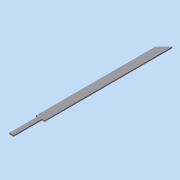
# Autodesk Inventor part: hoja1
Saved by Autodesk Inventor 2015 (Build 190159000, 159)
## iProperties
Created: 2017-10-03
Part Number: hoja1
Material: Generic
Document SubType Name: Modeling
Designer: macbook
Density: 1 g/cm^3
Appearance: Default
Author: macbook
Autodesk Inventor part; units mm, degrees
ref_plane "YZ Plane" through (0, 0, 0) normal (1, 0, 0) x (0, 1, 0)
ref_plane "XZ Plane" through (0, 0, 0) normal (0, 1, 0) x (-1, 0, 0)
ref_plane "XY Plane" through (0, 0, 0) normal (0, 0, 1) x (1, 0, 0)
sketch "Sketch1" plane through (0, 0, 0) normal (0, 0, 1) x (1, 0, 0)
  line L0 (0, 0) -> (18, 0)
  line L1 (18, 0) -> (18, 120)
  line L2 (18, 120) -> (29, 120)
  line L3 (0, 0) -> (0, 120)
  line L4 (0, 120) -> (-7, 120)
  line L5 (29, 120) -> (29, 660)
  line L6 (29, 120) -> (569, 120) construction
  line L7 (29, 660) -> (-7, 624)
  line L8 (29, 660) -> (79.9117, 660) construction
  line L9 (-7, 624) -> (-7, 120)
  dimension "d0" = 18
  dimension "d1" = 120
  dimension "d2" = 90
  dimension "d3" = 11
  dimension "d4" = 7
  dimension "d6" = 90
  dimension "d7" = 135
  constraints: 20 end point, 3 horizontal, 3 perpendicular, 2 equal length, 2 vertical
  measures "d0" distance of L0.start L0.end
  measures "d1" distance of L0.end L1.end
  measures "d2" angle of L1 L0
  measures "d3" distance of L1.end L2.end
  measures "d4" distance of L3.end L4.end
  measures "d6" angle of L6 L5
  measures "d7" angle of L7 L8
extrude "Extrusion1" add sketch "Sketch1" along normal blind 5.5
body "Solid1"
